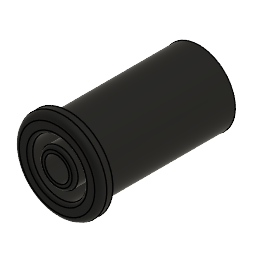
Bench power supply (Autodesk Fusion 360 archive; units mm, degrees)
design "BananaBlack"
Autodesk Fusion 360 part; units mm, degrees
sketch "Sketch1" plane through (0, 0, 0) normal (0, 1, 0) x (1, 0, 0)
  circle A0 centre (0, 0) radius 7.25
  dimension "d11" = 14.5
  constraint coincident A0.centre origin
  measures "d11" diameter of A0
extrude "Extrude1" add sketch "Sketch1" along normal blind 2
sketch "Sketch2" plane through (0, 2, 0) normal (0, 1, 0) x (-1, 0, 0)
  circle A0 centre (0, 0) radius 7.25
  circle A1 centre (0, 0) radius 6
  dimension "d14" = 12
  constraint concentric A0 A1
  measures "d14" diameter of A1
extrude "Extrude2" add sketch "Sketch2" along normal blind 21.5 contours A1
fillet "Fillet1" radius 1 1 edges at (-6.7594, 0, 2.6217)
sketch "Sketch4" plane through (0, 0, 0) normal (0, -1, 0) x (1, 0, 0)
  circle A0 centre (0, 0) radius 6.25
  circle A1 centre (0, 0) radius 2
  dimension "d26" = 4
  constraint coincident A0.centre A1.centre
  measures "d26" diameter of A1
extrude "Extrude4" cut sketch "Sketch4" against normal up to surface (23.5 mm away) contours A1
sketch "Sketch5" plane through (0, 0, 0) normal (0, -1, 0) x (1, 0, 0)
  circle A0 centre (0, 0) radius 2
  circle A1 centre (0, 0) radius 6.25
  circle A2 centre (0, 0) radius 3
  circle A3 centre (0, 0) radius 4.5
  dimension "d1" = 9
  dimension "d2" = 6
  constraint concentric A0 A2
  constraint coincident A0.centre A1.centre
  measures "d1" diameter of A3
  measures "d2" diameter of A2
extrude "Extrude5" cut sketch "Sketch5" against normal blind 10 contours A3
fillet "Fillet2" radius 0.5 2 edges at (-4.1955, 0, 1.6273) (-2.797, 0, -1.0848)
equation "d15 = 23.5 mm - 2 mm"

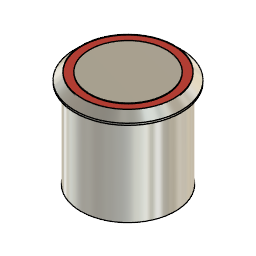
design "Anti-vandal"
Autodesk Fusion 360 part; units mm, degrees
sketch "Sketch1" plane through (0, 0, 0) normal (0, 0, 1) x (1, 0, 0)
  circle A0 centre (0, 0) radius 8
  dimension "d3" = 16
  constraint coincident A0.centre origin
  measures "d3" diameter of A0
extrude "Extrude1" add sketch "Sketch1" along normal blind 15
sketch "Sketch2" plane through (0, 0, 15) normal (0, 0, 1) x (-1, 0, 0)
  circle A0 centre (0, 0) radius 8
  circle A1 centre (0, 0) radius 9
  dimension "d4" = 18
  constraint coincident A0.centre A1.centre
  measures "d4" diameter of A1
extrude "Extrude2" add sketch "Sketch2" along normal blind 1.5 contours A0 | A1
chamfer "Chamfer1" distance 1.2 angle 45 1 edges at (8.3909, 3.2545, 16.5)
sketch "Sketch3" plane through (0, 0, 16.5) normal (0, 0, 1) x (-1, 0, 0)
  circle A0 centre (0, 0) radius 7.8
  circle A1 centre (0, 0) radius 6.5
  dimension "d10" = 13
  constraint concentric A0 A1
  measures "d10" diameter of A1
extrude "Extrude3" cut sketch "Sketch3" against normal blind 0.1

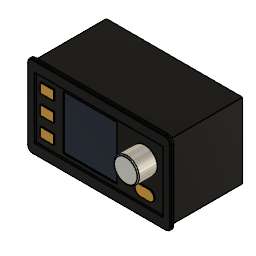
design "DPS5005"
Autodesk Fusion 360 part; units mm, degrees
sketch "Sketch7" plane through (0, 0, 0) normal (0, -1, 0) x (1, 0, 0)
  line L0 (-35.442, 76.9329) -> (35.558, 76.9329)
  line L1 (-35.442, 37.9329) -> (-35.442, 76.9329)
  line L2 (35.558, 37.9329) -> (-35.442, 37.9329)
  line L3 (35.558, 76.9329) -> (35.558, 37.9329)
extrude "Extrude2" add sketch "Sketch7" against normal blind 38
sketch "Sketch8" plane through (0, 0, 0) normal (0, -1, 0) x (1, 0, 0)
  line L0 (35.558, 76.9329) -> (-35.442, 76.9329)
  line L1 (-35.442, 76.9329) -> (-35.442, 37.9329)
  line L2 (-35.442, 37.9329) -> (35.558, 37.9329)
  line L3 (35.558, 37.9329) -> (35.558, 76.9329)
  line L4 (-37.442, 35.9329) -> (37.558, 35.9329)
  line L5 (37.558, 35.9329) -> (37.558, 78.9329)
  line L6 (37.558, 78.9329) -> (-37.442, 78.9329)
  line L7 (-37.442, 78.9329) -> (-37.442, 35.9329)
  dimension "d62" = 2
extrude "Extrude3" add sketch "Sketch8" along normal blind 1.5 contours L0 L1 L2 L3 | L4 L5 L6 L7
fillet "Fillet1" radius 3 4 edges at (-37.442, -0.75, 78.9329) (-37.442, -0.75, 35.9329) (37.558, -0.75, 35.9329) (37.558, -0.75, 78.9329)
fillet "Fillet2" radius 0.5 1 faces at (11.558, -1.5, 64.5996)
sketch "Sketch9" plane through (0, -1.5, 0) normal (0, -1, 0) x (1, 0, 0)
  arc A0 (37.058, 75.9329) -> (34.558, 78.4329) centre (34.558, 75.9329) ccw
  line L0 (34.558, 78.4329) -> (-34.442, 78.4329)
  arc A1 (-34.442, 78.4329) -> (-36.942, 75.9329) centre (-34.442, 75.9329) ccw
  line L1 (-36.942, 75.9329) -> (-36.942, 38.9329)
  arc A2 (-36.942, 38.9329) -> (-34.442, 36.4329) centre (-34.442, 38.9329) ccw
  line L2 (-34.442, 36.4329) -> (34.558, 36.4329)
  arc A3 (34.558, 36.4329) -> (37.058, 38.9329) centre (34.558, 38.9329) ccw
  line L3 (37.058, 38.9329) -> (37.058, 75.9329)
  line L4 (0.058, 78.4329) -> (0.058, 36.4329) construction
  line L5 (33.558, 73.4329) -> (-33.442, 73.4329)
  line L6 (-33.442, 73.4329) -> (-33.442, 41.4329)
  line L7 (-33.442, 41.4329) -> (33.558, 41.4329)
  line L8 (33.558, 41.4329) -> (33.558, 73.4329)
  line L9 (33.558, 73.4329) -> (-33.442, 41.4329) construction
  line L10 (-33.442, 73.4329) -> (33.558, 41.4329) construction
  point P0 (0.058, 57.4329)
  dimension "d5" = 67
  dimension "d6" = 32
  constraint midpoint L0 L4.start
  constraint midpoint L2 L4.end
  constraint horizontal L5
  constraint perpendicular L5 L6
  constraint parallel L5 L7
  constraint parallel L6 L8
  constraint coincident L9 P0
  constraint coincident L10 P0
  constraint midpoint L4 P0
  measures "d5" distance of L5.start L5.end
  measures "d6" distance of L5.start L7.end
extrude "Extrude4" cut sketch "Sketch9" against normal blind 1 contours L5 L6 L7 L8
sketch "Sketch10" plane through (0, -0.5, 0) normal (0, -1, 0) x (1, 0, 0)
  line L0 (33.558, 41.4329) -> (33.558, 73.4329)
  line L1 (33.558, 73.4329) -> (-33.442, 73.4329)
  line L2 (-33.442, 73.4329) -> (-33.442, 41.4329)
  line L3 (-33.442, 41.4329) -> (33.558, 41.4329)
  line L4 (-19.442, 71.4329) -> (8.558, 71.4329)
  line L5 (8.558, 71.4329) -> (8.558, 43.4329)
  line L6 (8.558, 43.4329) -> (-19.442, 43.4329)
  line L7 (-19.442, 43.4329) -> (-19.442, 71.4329)
  dimension "d9" = 28
  dimension "d10" = 28
  dimension "d11" = 14
  dimension "d12" = 2
  constraint horizontal L4
  constraint vertical L5
  constraint horizontal L6
  constraint vertical L7
  measures "d9" distance of L4.start L4.end
  measures "d10" distance of L4.end L5.end
  measures "d11" distance of L2 L7
  measures "d12" distance of L1 L4
extrude "Extrude5" cut sketch "Sketch10" against normal blind 0.5 contours L4 L5 L6 L7
sketch "Sketch11" plane through (0, -0.5, 0) normal (0, -1, 0) x (1, 0, 0)
  line L0 (8.558, 71.4329) -> (8.558, 43.4329)
  line L1 (8.558, 43.4329) -> (-19.442, 43.4329)
  line L2 (-19.442, 43.4329) -> (-19.442, 71.4329)
  line L3 (-19.442, 71.4329) -> (8.558, 71.4329)
  line L4 (33.558, 41.4329) -> (33.558, 73.4329)
  line L5 (33.558, 73.4329) -> (-33.442, 73.4329)
  line L6 (-33.442, 73.4329) -> (-33.442, 41.4329)
  line L7 (-33.442, 41.4329) -> (33.558, 41.4329)
  line L8 (-27.442, 73.4329) -> (-27.442, 41.4329) construction
  line L9 (-23.942, 59.9329) -> (-30.942, 59.9329)
  line L10 (-30.942, 59.9329) -> (-30.942, 54.9329)
  line L11 (-30.942, 54.9329) -> (-23.942, 54.9329)
  line L12 (-23.942, 54.9329) -> (-23.942, 59.9329)
  line L13 (-23.942, 59.9329) -> (-30.942, 54.9329) construction
  line L14 (-30.942, 59.9329) -> (-23.942, 54.9329) construction
  line L15 (-23.942, 69.9329) -> (-30.942, 69.9329)
  line L16 (-30.942, 69.9329) -> (-30.942, 64.9329)
  line L17 (-30.942, 64.9329) -> (-23.942, 64.9329)
  line L18 (-23.942, 64.9329) -> (-23.942, 69.9329)
  line L19 (-23.942, 69.9329) -> (-30.942, 64.9329) construction
  line L20 (-30.942, 69.9329) -> (-23.942, 64.9329) construction
  line L21 (-23.942, 49.9329) -> (-30.942, 49.9329)
  line L22 (-30.942, 49.9329) -> (-30.942, 44.9329)
  line L23 (-30.942, 44.9329) -> (-23.942, 44.9329)
  line L24 (-23.942, 44.9329) -> (-23.942, 49.9329)
  line L25 (-23.942, 49.9329) -> (-30.942, 44.9329) construction
  line L26 (-30.942, 49.9329) -> (-23.942, 44.9329) construction
  line L27 (21.1522, 44.4173) -> (25.6596, 44.4173)
  arc A0 (25.6596, 44.4173) -> (25.6596, 49.9237) centre (25.6596, 47.1705) ccw
  line L28 (25.6596, 49.9237) -> (21.1522, 49.9237)
  arc A1 (21.1522, 49.9237) -> (21.1522, 44.4173) centre (21.1522, 47.1705) ccw
  line L29 (21.1522, 47.1705) -> (25.6596, 47.1705) construction
  point P0 (-27.442, 57.4329)
  point P1 (-27.442, 67.4329)
  point P2 (-27.442, 47.4329)
  dimension "d15" = 7
  dimension "d16" = 5
  dimension "d19" = 7
  dimension "d20" = 5
  dimension "d21" = 7
  dimension "d22" = 5
  dimension "d23" = 6
  dimension "d24" = 5
  dimension "d25" = 5
  constraint coincident L5 L8.start
  constraint coincident L7 L8.end
  constraint perpendicular L7 L8
  constraint horizontal L9
  constraint perpendicular L9 L10
  constraint parallel L9 L11
  constraint parallel L10 L12
  constraint coincident L13 P0
  constraint coincident L14 P0
  constraint midpoint L8 P0
  constraint horizontal L15
  constraint perpendicular L15 L16
  constraint parallel L15 L17
  constraint parallel L16 L18
  constraint coincident L19 P1
  constraint coincident L20 P1
  constraint horizontal L21
  constraint perpendicular L21 L22
  constraint parallel L21 L23
  constraint parallel L22 L24
  constraint coincident L25 P2
  constraint coincident L26 P2
  constraint coincident L8 P2
  constraint coincident L8 P1
  constraint tangent L27 A0
  constraint tangent A0 L28
  constraint parallel L27 L28
  constraint tangent L28 A1
  constraint tangent L27 A1
  constraint horizontal L29
  measures "d15" distance of L9.start L9.end
  measures "d16" distance of L9.start L11.end
  measures "d19" distance of L21.start L21.end
  measures "d20" distance of L21.start L23.end
  measures "d21" distance of L15.start L15.end
  measures "d22" distance of L15.start L17.end
  measures "d23" distance of L6 L8
  measures "d24" distance of L9 L17
  measures "d25" distance of L11 L21
extrude "Extrude6" add sketch "Sketch11" along normal blind 0.5 contours L9 L10 L11 L12 | L15 L16 L17 L18 | L21 L22 L23 L24 | L27 A0 L28 A1
sketch "Sketch12" plane through (0, -0.5, 0) normal (0, -1, 0) x (1, 0, 0)
  line L0 (-23.942, 64.9329) -> (-30.942, 64.9329)
  line L1 (-30.942, 64.9329) -> (-30.942, 69.9329)
  line L2 (-30.942, 69.9329) -> (-23.942, 69.9329)
  line L3 (-23.942, 69.9329) -> (-23.942, 64.9329)
  line L4 (-23.942, 44.9329) -> (-30.942, 44.9329)
  line L5 (-30.942, 44.9329) -> (-30.942, 49.9329)
  line L6 (-30.942, 49.9329) -> (-23.942, 49.9329)
  line L7 (-23.942, 49.9329) -> (-23.942, 44.9329)
  line L8 (-23.942, 54.9329) -> (-30.942, 54.9329)
  line L9 (-30.942, 54.9329) -> (-30.942, 59.9329)
  line L10 (-30.942, 59.9329) -> (-23.942, 59.9329)
  line L11 (-23.942, 59.9329) -> (-23.942, 54.9329)
  line L12 (8.558, 71.4329) -> (8.558, 43.4329)
  line L13 (8.558, 43.4329) -> (-19.442, 43.4329)
  line L14 (-19.442, 43.4329) -> (-19.442, 71.4329)
  line L15 (-19.442, 71.4329) -> (8.558, 71.4329)
  line L16 (33.558, 41.4329) -> (33.558, 73.4329)
  line L17 (33.558, 73.4329) -> (-33.442, 73.4329)
  line L18 (-33.442, 73.4329) -> (-33.442, 41.4329)
  line L19 (-33.442, 41.4329) -> (33.558, 41.4329)
  line L20 (23.1489, 73.4329) -> (23.1489, 41.4329) construction
  circle A0 centre (23.1489, 61.9329) radius 6.5
  line L21 (21.1522, 49.9237) -> (25.6596, 49.9237)
  arc A1 (25.6596, 44.4173) -> (25.6596, 49.9237) centre (25.6596, 47.1705) ccw
  line L22 (25.6596, 44.4173) -> (21.1522, 44.4173)
  arc A2 (21.1522, 49.9237) -> (21.1522, 44.4173) centre (21.1522, 47.1705) ccw
  dimension "d26" = 13
  dimension "d27" = 11.5
  constraint coincident L17 L20.start
  constraint coincident L19 L20.end
  constraint perpendicular L19 L20
  constraint coincident L20 A0.centre
  measures "d26" diameter of A0
  measures "d27" distance of L17 A0.centre
extrude "Extrude7" add sketch "Sketch12" along normal blind 10 contours A0
fillet "Fillet3" radius 0.5 1 edges at (17.0888, -10.5, 59.5824)

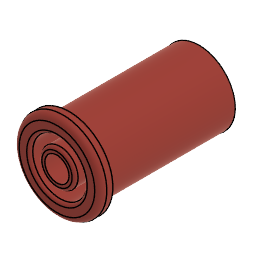
design "BananaRed"
Autodesk Fusion 360 part; units mm, degrees
sketch "Sketch1" plane through (0, 0, 0) normal (0, 1, 0) x (1, 0, 0)
  circle A0 centre (0, 0) radius 7.25
  dimension "d11" = 14.5
  constraint coincident A0.centre origin
  measures "d11" diameter of A0
extrude "Extrude1" add sketch "Sketch1" along normal blind 2
sketch "Sketch2" plane through (0, 2, 0) normal (0, 1, 0) x (-1, 0, 0)
  circle A0 centre (0, 0) radius 7.25
  circle A1 centre (0, 0) radius 6
  dimension "d14" = 12
  constraint concentric A0 A1
  measures "d14" diameter of A1
extrude "Extrude2" add sketch "Sketch2" along normal blind 21.5 contours A1
fillet "Fillet1" radius 1 1 edges at (-6.7594, 0, 2.6217)
sketch "Sketch4" plane through (0, 0, 0) normal (0, -1, 0) x (1, 0, 0)
  circle A0 centre (0, 0) radius 6.25
  circle A1 centre (0, 0) radius 2
  dimension "d26" = 4
  constraint coincident A0.centre A1.centre
  measures "d26" diameter of A1
extrude "Extrude4" cut sketch "Sketch4" against normal up to surface (23.5 mm away) contours A1
sketch "Sketch5" plane through (0, 0, 0) normal (0, -1, 0) x (1, 0, 0)
  circle A0 centre (0, 0) radius 2
  circle A1 centre (0, 0) radius 6.25
  circle A2 centre (0, 0) radius 3
  circle A3 centre (0, 0) radius 4.5
  dimension "d1" = 9
  dimension "d2" = 6
  constraint concentric A0 A2
  constraint coincident A0.centre A1.centre
  measures "d1" diameter of A3
  measures "d2" diameter of A2
extrude "Extrude5" cut sketch "Sketch5" against normal blind 10 contours A3
fillet "Fillet2" radius 0.5 2 edges at (-4.1955, 0, 1.6273) (-2.797, 0, -1.0848)
equation "d15 = 23.5 mm - 2 mm"

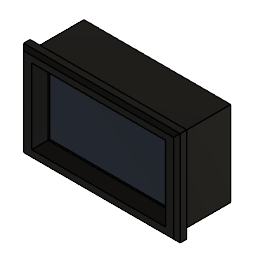
design "Meter"
Autodesk Fusion 360 part; units mm, degrees
sketch "Sketch1" plane through (0, 0, 0) normal (0, 1, 0) x (1, 0, 0)
  line L0 (24, 35.5) -> (-24, 35.5)
  line L1 (-24, 35.5) -> (-24, 64.5)
  line L2 (-24, 64.5) -> (24, 64.5)
  line L3 (24, 64.5) -> (24, 35.5)
  line L4 (24, 35.5) -> (-24, 64.5) construction
  line L5 (-24, 35.5) -> (24, 64.5) construction
  point P0 (0, 50)
  dimension "d33" = 48
  dimension "d34" = 29
  constraint horizontal L0
  constraint perpendicular L0 L1
  constraint parallel L0 L2
  constraint parallel L1 L3
  constraint coincident L4 P0
  constraint coincident L5 P0
  measures "d33" distance of L0.start L0.end
  measures "d34" distance of L0.start L2.end
extrude "Extrude1" add sketch "Sketch1" against normal blind 3
sketch "Sketch2" plane through (0, 0, 0) normal (0, 1, 0) x (-1, 0, 0)
  line L0 (-24, -64.5) -> (24, -64.5)
  line L1 (24, -64.5) -> (24, -35.5)
  line L2 (24, -35.5) -> (-24, -35.5)
  line L3 (-24, -35.5) -> (-24, -64.5)
  line L4 (22.5, -37) -> (-22.5, -37)
  line L5 (-22.5, -37) -> (-22.5, -63)
  line L6 (-22.5, -63) -> (22.5, -63)
  line L7 (22.5, -63) -> (22.5, -37)
  line L8 (22.5, -37) -> (-22.5, -63) construction
  line L9 (-22.5, -37) -> (22.5, -63) construction
  point P0 (0, -50)
  dimension "d37" = 45
  dimension "d38" = 26
  constraint horizontal L4
  constraint perpendicular L4 L5
  constraint parallel L4 L6
  constraint parallel L5 L7
  constraint coincident L8 P0
  constraint coincident L9 P0
  measures "d37" distance of L4.start L4.end
  measures "d38" distance of L4.end L5.end
extrude "Extrude2" add sketch "Sketch2" along normal blind 15 contours L4 L5 L6 L7
chamfer "Chamfer1" distance 1 angle 45 1 faces at (8, -3, -45.1667)
sketch "Sketch3" plane through (0, -3, 0) normal (0, -1, 0) x (1, 0, 0)
  line L0 (23, -36.5) -> (-23, -36.5)
  line L1 (-23, -36.5) -> (-23, -63.5)
  line L2 (-23, -63.5) -> (23, -63.5)
  line L3 (23, -63.5) -> (23, -36.5)
  line L4 (0, -36.5) -> (0, -63.5) construction
  line L5 (18, -41) -> (-18, -41)
  line L6 (-18, -41) -> (-18, -59)
  line L7 (-18, -59) -> (18, -59)
  line L8 (18, -59) -> (18, -41)
  line L9 (18, -41) -> (-18, -59) construction
  line L10 (-18, -41) -> (18, -59) construction
  point P0 (0, -50)
  dimension "d1" = 36
  dimension "d2" = 18
  constraint midpoint L0 L4.start
  constraint midpoint L2 L4.end
  constraint horizontal L5
  constraint perpendicular L5 L6
  constraint parallel L5 L7
  constraint parallel L6 L8
  constraint coincident L9 P0
  constraint coincident L10 P0
  constraint midpoint L4 P0
  measures "d1" distance of L5.start L5.end
  measures "d2" distance of L5.start L7.end
extrude "Extrude3" cut sketch "Sketch3" against normal blind 3 contours L5 L6 L7 L8
chamfer "Chamfer2" distance 2.5 angle 45 4 edges at (0, -3, -41) (-18, -3, -50) (0, -3, -59) (18, -3, -50)
